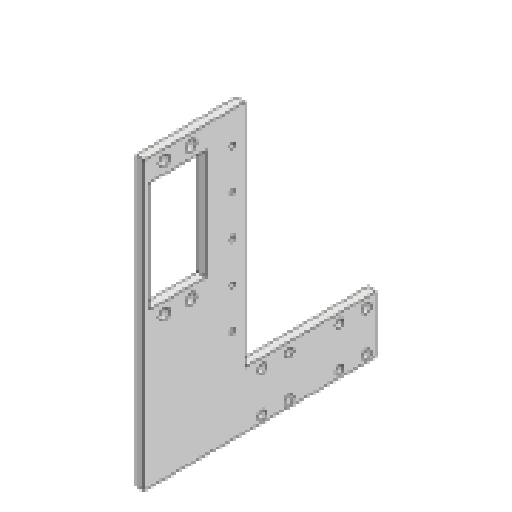
# Autodesk Inventor part: LinearSlidePlate
Saved by Autodesk Inventor 2023 (Build 270158000, 158)
## iProperties
Created: 2022-10-31
Part Number: LinearSlidePlate
Material: Generic
Document SubType Name: Modeling
Designer: deli
Density: 1 g/cm^3
Appearance: Default
Author: deli
Autodesk Inventor part; units mm, degrees
ref_plane "YZ Plane" through (0, 0, 0) normal (1, 0, 0) x (0, 1, 0)
ref_plane "XZ Plane" through (0, 0, 0) normal (0, 1, 0) x (-1, 0, 0)
ref_plane "XY Plane" through (0, 0, 0) normal (0, 0, 1) x (1, 0, 0)
sketch "Sketch1" plane through (0, 0, 0) normal (1, 0, 0) x (0, 1, 0)
  circle A0 centre (-28.0038, 5.7897) radius 1.6
  circle A1 centre (-28.0038, -4.2103) radius 1.6
  circle A2 centre (-43.0038, 5.7897) radius 1.6
  circle A3 centre (-43.0038, -4.2103) radius 1.6
  line L0 (-28.0038, 5.7897) -> (-28.0038, -4.2103) construction
  line L1 (-28.0038, -4.2103) -> (-43.0038, -4.2103) construction
  line L2 (-43.0038, -4.2103) -> (-43.0038, 5.7897) construction
  line L3 (-43.0038, 5.7897) -> (-28.0038, 5.7897) construction
  line L4 (61.2962, 49.7897) -> (-45.5038, 49.7897)
  line L5 (-45.5038, 49.7897) -> (-45.5038, -36.7103)
  line L6 (-45.5038, -36.7103) -> (-24.4038, -36.7103)
  line L7 (61.2962, 12.2897) -> (61.2962, 49.7897)
  circle A4 centre (7.6962, 32.2897) radius 2
  circle A5 centre (7.6962, 42.2897) radius 2
  circle A6 centre (57.2962, 32.2897) radius 2
  circle A7 centre (57.2962, 42.2897) radius 2
  line L8 (7.6962, 32.2897) -> (7.6962, 42.2897) construction
  line L9 (7.6962, 42.2897) -> (57.2962, 42.2897) construction
  line L10 (57.2962, 42.2897) -> (57.2962, 32.2897) construction
  line L11 (57.2962, 32.2897) -> (7.6962, 32.2897) construction
  line L12 (11.9962, 26.7897) -> (52.9962, 26.7897)
  line L13 (52.9962, 26.7897) -> (52.9962, 47.7897)
  line L14 (52.9962, 47.7897) -> (11.9962, 47.7897)
  line L15 (11.9962, 47.7897) -> (11.9962, 26.7897)
  circle A8 centre (-10.5038, 16.7897) radius 1
  circle A9 centre (4.4962, 16.7897) radius 1
  circle A10 centre (19.4962, 16.7897) radius 1
  circle A11 centre (34.4962, 16.7897) radius 1
  line L16 (34.4962, 16.7897) -> (-45.5038, 16.7897) construction
  circle A12 centre (-28.0038, -23.1103) radius 1.6
  circle A13 centre (-28.0038, -33.1103) radius 1.6
  circle A14 centre (-43.0038, -23.1103) radius 1.6
  circle A15 centre (-43.0038, -33.1103) radius 1.6
  line L17 (-28.0038, -23.1103) -> (-28.0038, -33.1103) construction
  line L18 (-28.0038, -33.1103) -> (-43.0038, -33.1103) construction
  line L19 (-43.0038, -33.1103) -> (-43.0038, -23.1103) construction
  line L20 (-43.0038, -23.1103) -> (-28.0038, -23.1103) construction
  line L21 (61.2962, 12.2897) -> (-24.4038, 12.2897)
  line L22 (-24.4038, 12.2897) -> (-24.4038, -36.7103)
  circle A16 centre (49.4962, 16.7897) radius 1
  point P0 (0, 0)
  dimension "d0" = 3.2
  dimension "d1" = 10
  dimension "d2" = 15
  dimension "d9" = 4
  dimension "d10" = 10
  dimension "d11" = 49.6
  dimension "d12" = 21
  dimension "d13" = 41
  dimension "d14" = 5.5
  dimension "d15" = 4.3
  dimension "d21" = 2
  dimension "d25" = 15
  dimension "d32" = 15
  dimension "d33" = 15
  dimension "d36" = 2
  dimension "d37" = 35
  dimension "d38" = 10
  dimension "d39" = 2
  dimension "d40" = 2.5
  dimension "d41" = 10
  dimension "d42" = 40
  dimension "d44" = 3.2
  dimension "d45" = 10
  dimension "d46" = 15
  dimension "d47" = 18.9
  dimension "d48" = 2
  dimension "d50" = 2
  dimension "d51" = 3.5
  dimension "d52" = 15
  constraints: 46 end point, 17 centre point, 13 equal radius, 13 perpendicular, 5 parallel, 5 point on line, 2 horizontal, 2 vertical, 1 collinear
  measures "d0" diameter of A0
  measures "d1" distance of L0.start L0.end
  measures "d2" distance of L2.end L0.start
  measures "d9" diameter of A4
  measures "d10" distance of L8.start L8.end
  measures "d11" distance of L10.end L8.start
  measures "d12" distance of L14.end L12.start
  measures "d13" distance of L12.start L12.end
  measures "d14" distance between parallel lines of L11 L12
  measures "d15" distance between parallel lines of L8 L15
  measures "d21" diameter of A8
  measures "d25" distance of A8.centre A9.centre
  measures "d32" distance of A10.centre A9.centre
  measures "d33" distance of L16.start A10.centre
  measures "d36" distance edge to line of A7 L7
  measures "d37" distance from line of L5 A8.centre
  measures "d38" distance from line of A10.centre L12
  measures "d39" distance between parallel lines of L4 L14
  measures "d40" distance between parallel lines of L5 L2
  measures "d41" distance edge to line of A8 L3
  measures "d42" distance between parallel lines of L0 L15
  measures "d44" diameter of A12
  measures "d45" distance of L17.start L17.end
  measures "d46" distance of L20.start L17.start
  measures "d47" distance between parallel lines of L20 L1
  measures "d48" distance edge to line of A13 L6
  measures "d50" distance edge to line of A13 L22
  measures "d51" distance edge to line of A11 L21
  measures "d52" distance of L16.start A16.centre
extrude "Extrusion1" add sketch "Sketch1" along normal blind 3.175
equation "\"d14\" = -0.5 * d10 + 0.5 * d12"
equation "\"d15\" = -0.5 * d13 + 0.5 * d11"
equation "\"d32\" = d25"
equation "\"d33\" = d32"
body "Solid1"
